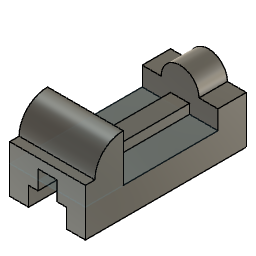
Shape 2_ (Autodesk Fusion 360 design; units mm, degrees)
Autodesk Fusion 360 part; units mm, degrees
sketch "Sketch1" plane through (0, 0, 0) normal (0, 0, 1) x (1, 0, 0)
  line L0 (0, 0) -> (-80, 0)
  line L1 (-80, 0) -> (-80, 170)
  line L2 (-80, 170) -> (0, 170)
  line L3 (0, 170) -> (0, 0)
  dimension "d1" = 80
  dimension "d2" = 170
  constraint horizontal L0
  constraint vertical L1
  constraint horizontal L2
  constraint vertical L3
  constraint coincident L0.start L3.end
  measures "d1" distance of L0.start L0.end
  measures "d2" distance of L0.start L2.end
extrude "Extrude1" add sketch "Sketch1" along normal blind 30 makes body 1
sketch "Sketch2" plane through (0, 0, 30) normal (0, 0, 1) x (-1, 0, 0)
  line L0 (0, -170) -> (80, -170)
  line L1 (80, -170) -> (80, 0)
  line L2 (80, 0) -> (0, 0)
  line L3 (0, 0) -> (0, -170)
  line L4 (80, -170) -> (0, -170)
  line L5 (0, -170) -> (0, -140)
  line L6 (0, -140) -> (80, -140)
  line L7 (80, -140) -> (80, -170)
  dimension "d5" = 30
  constraint horizontal L4
  constraint vertical L5
  constraint horizontal L6
  constraint vertical L7
  constraint coincident L0.end L1.start
  measures "d5" distance of L0.end L6.end
extrude "Extrude2" add sketch "Sketch2" along normal blind 20 contours L0 L1 L3 L4 L5 L6 L7 bodies 1
sketch "Sketch3" plane through (0, 140, 0) normal (0, -1, 0) x (1, 0, 0)
  line L0 (-80, 30) -> (0, 30)
  line L1 (0, 30) -> (0, 50)
  line L2 (0, 50) -> (-80, 50)
  line L3 (-80, 50) -> (-80, 30)
  arc A0 (-20, 50) -> (-60, 50) centre (-40, 50) ccw
  dimension "d8" = 20
  constraint coincident L2 A0.start
  constraint midpoint L2 A0.centre
  measures "d8" radius of A0
extrude "Extrude3" add sketch "Sketch3" against normal blind 30 contours L2 A0 bodies 1
sketch "Sketch4" plane through (0, 0, 30) normal (0, 0, 1) x (-1, 0, 0)
  line L0 (0, -140) -> (80, -140)
  line L1 (80, -140) -> (80, 0)
  line L2 (80, 0) -> (0, 0)
  line L3 (0, 0) -> (0, -140)
sketch "Sketch5" plane through (0, 0, 30) normal (0, 0, 1) x (-1, 0, 0)
  line L0 (80, 0) -> (0, 0)
  line L1 (0, 0) -> (0, -40)
  line L2 (0, -40) -> (80, -40)
  line L3 (80, -40) -> (80, 0)
  dimension "d11" = 40
  constraint horizontal L0
  constraint vertical L1
  constraint horizontal L2
  constraint vertical L3
  measures "d11" distance of L0.start L2.end
extrude "Extrude4" add sketch "Sketch5" along normal blind 20 bodies 1
sketch "Sketch6" plane through (0, 0, 0) normal (1, 0, 0) x (0, 1, 0)
  line L0 (0, 0) -> (170, 0)
  line L1 (170, 0) -> (170, 50)
  line L2 (170, 50) -> (140, 50)
  line L3 (140, 50) -> (140, 30)
  line L4 (140, 30) -> (40, 30)
  line L5 (40, 30) -> (40, 50)
  line L6 (40, 50) -> (0, 50)
  line L7 (0, 50) -> (0, 0)
  arc A0 (40, 80) -> (10, 50) centre (40, 50) ccw
  line L8 (40, 80) -> (40, 50)
  dimension "d14" = 30
  constraint coincident L5.end L6.start
  constraint perpendicular L6 L8
  measures "d14" radius of A0
extrude "Extrude5" add sketch "Sketch6" against normal blind 80 contours L6 A0 L8 bodies 1
sketch "Sketch7" plane through (0, 0, 30) normal (0, 0, 1) x (1, 0, 0)
  line L0 (-40, 140) -> (-50, 140)
  line L1 (-50, 140) -> (-50, 40)
  line L2 (-50, 40) -> (-40, 40)
  line L3 (-40, 140) -> (-30, 140)
  line L4 (-30, 140) -> (-30, 40)
  line L5 (-30, 40) -> (-40, 40)
  constraint horizontal L0
  constraint vertical L1
  constraint horizontal L2
  constraint horizontal L3
  constraint vertical L4
  constraint horizontal L5
extrude "Extrude6" add sketch "Sketch7" along normal blind 10 bodies 1
sketch "Sketch8" plane through (0, 0, 0) normal (0, 0, -1) x (1, 0, 0)
  line L0 (-80, -170) -> (0, -170)
  line L1 (0, -170) -> (0, 0)
  line L2 (0, 0) -> (-80, 0)
  line L3 (-80, 0) -> (-80, -170)
  line L4 (-40, 0) -> (-60, 0)
  line L5 (-60, 0) -> (-60, -170)
  line L6 (-60, -170) -> (-40, -170)
  line L7 (-40, 0) -> (-20, 0)
  line L8 (-20, 0) -> (-20, -170)
  line L9 (-20, -170) -> (-40, -170)
  dimension "d20" = 20
  constraint horizontal L4
  constraint vertical L5
  constraint horizontal L6
  constraint midpoint L2 L4.start
  constraint horizontal L7
  constraint vertical L8
  constraint horizontal L9
  measures "d20" distance of L4.start L4.end
extrude "Extrude7" cut sketch "Sketch8" against normal blind 20 contours L0 L2 L4 L5 L6 L7 L8 L9 bodies 1
sketch "Sketch9" plane through (0, 0, 20) normal (0, 0, -1) x (1, 0, 0)
  line L0 (-20, 0) -> (-60, 0)
  line L1 (-60, 0) -> (-60, -170)
  line L2 (-60, -170) -> (-20, -170)
  line L3 (-20, -170) -> (-20, 0)
  line L4 (-40, 0) -> (-50, 0)
  line L5 (-50, 0) -> (-50, -170)
  line L6 (-50, -170) -> (-40, -170)
  line L7 (-40, 0) -> (-30, 0)
  line L8 (-30, 0) -> (-30, -170)
  line L9 (-30, -170) -> (-40, -170)
  constraint horizontal L4
  constraint vertical L5
  constraint horizontal L6
  constraint coincident L2 L5.end
  constraint midpoint L0 L4.start
  constraint horizontal L7
  constraint vertical L8
  constraint horizontal L9
  constraint coincident L2 L8.end
extrude "Extrude8" cut sketch "Sketch9" against normal blind 20 contours L0 L2 L4 L5 L6 L7 L8 L9 bodies 1
sketch "Sketch10" plane through (0, 0, 30) normal (0, 0, 1) x (1, 0, 0)
  line L0 (-50, 40) -> (-30, 40)
  line L1 (-30, 40) -> (-30, 140)
  line L2 (-30, 140) -> (-50, 140)
  line L3 (-50, 140) -> (-50, 40)
  constraint horizontal L0
  constraint vertical L1
  constraint horizontal L2
  constraint vertical L3
extrude "Extrude9" add sketch "Sketch10" along normal blind 10 separate body makes body 2
